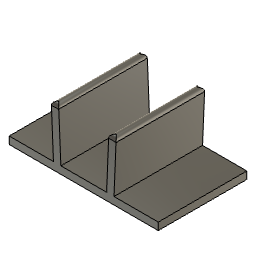
Pipette_Holder_before_LPS_injection v1 (Autodesk Fusion 360 design; units mm, degrees)
Autodesk Fusion 360 part; units mm, degrees
note: some values were not read from the file. Chosen so that the rebuilt part matches the saved one: which bodies a step acts on; which face or edge a step refers to.
sketch "Sketch1" plane through (0, 0, 0) normal (0, 0, 1) x (1, 0, 0)
  line L0 (0, 0) -> (31, 0)
  line L1 (31, 0) -> (31, 60)
  line L2 (31, 60) -> (0, 60)
  line L3 (0, 60) -> (0, 0)
  line L4 (0, 0, 0) -> (0, 0, 35)
  line L5 (0, 0, 35) -> (32.5, 0, 35)
  line L6 (0, 0, 35) -> (-1.5, 0, 35)
  line L7 (-1.5, 0, 35) -> (32.5, 0, 35)
  line L8 (32.5, 0, 35) -> (32.5, 60, 35)
  line L9 (32.5, 60, 35) -> (-1.5, 60, 35)
  line L10 (-1.5, 60, 35) -> (-1.5, 0, 35)
  dimension "d1" = 31
  dimension "d2" = 60
  dimension "d3" = 35
  dimension "d4" = 32.5
  dimension "d5" = 1.5
  dimension "d6" = 60
  constraint horizontal L0
  constraint vertical L1
  constraint horizontal L2
  constraint vertical L3
  constraint coincident L0.start L3.end
  measures "d1" distance of L0.start L0.end
  measures "d2" distance of L0.start L2.end
  measures "d3" distance of L0.start L3.end
sketch "Sketch1 (curves 35 mm off its plane)" plane through (0, 0, 35) normal (0, 0, 1) x (1, 0, 0)
  line L0 (0, 0) -> (32.5, 0)
  line L1 (0, 0) -> (-1.5, 0)
  line L2 (-1.5, 0) -> (32.5, 0)
  line L3 (32.5, 0) -> (32.5, 60)
  line L4 (32.5, 60) -> (-1.5, 60)
  line L5 (-1.5, 60) -> (-1.5, 0)
loft "Loft1" add profiles "Sketch1", "Sketch1 (curves 35 mm off its plane)" section 1 section 2 makes body 1
extrude "Extrude1" add 1 faces at (-0.5, 40, 11.6667) along direction (-0.999083, 0, -0.042818) blind 5 separate body on bodies 1 makes body 2
extrude "Extrude2" add 1 faces at (-1.6651, 40, -0.0714) along direction (0.042818, 0, -0.999083) blind 30 on bodies 2 bodies 2
extrude "Extrude3" cut 1 faces at (10.3333, 40, 0) along direction (0, 0, -1) blind 35 on bodies 1 bodies 2
extrude "Extrude4" cut 1 faces at (0, 40, -10.0092) along direction (-1, 0, 0) blind 10 on bodies 2 bodies 2 makes body 3 at (-0.5, 40, 11.6667)
extrude "Extrude5" add 1 faces at (31.5, 40, 11.6667) along direction (0.999083, 0, -0.042818) blind 5 separate body on bodies 1 makes body 4
extrude "Extrude6" add 1 faces at (32.6651, 20, -0.0714) along direction (-0.042818, 0, -0.999083) blind 20 on bodies 4 bodies 4
extrude "Extrude7" cut 1 faces at (10.3333, 40, 0) along direction (0, 0, -1) blind 30 on bodies 1 bodies 4
extrude "Extrude8" cut 1 faces at (31, 20, -6.6728) along direction (1, 0, 0) blind 20 on bodies 4 bodies 4 makes body 5 at (31.5, 40, 11.6667)
extrude "Extrude9" add 3 faces at (32.6682, 20, 0) (10.3333, 40, 0) (-1.6682, 40, 0) along direction (0, 0, -1) blind 5 on bodies 1 3 5 bodies 5 3
extrude "Extrude10" add 1 faces at (-5.0046, 20, -1.6667) along direction (-1, 0, 0) blind 30 on bodies 5 bodies 5
extrude "Extrude11" add 1 faces at (36.0046, 40, -1.6667) along direction (1, 0, 0) blind 30 on bodies 5 bodies 5
fillet "Fillet1" radius 2.5 4 edges at (34.9977, 60, 34.893) (34.9977, 0, 34.893) (37.4954, 30, 34.7859) (32.5, 30, 35) on bodies 5
fillet "Fillet2" radius 2.5 4 edges at (-3.9977, 60, 34.893) (-1.5, 30, 35) (-3.9977, 0, 34.893) (-6.4954, 30, 34.7859) on bodies 5
hidden bodies 1 2 4
